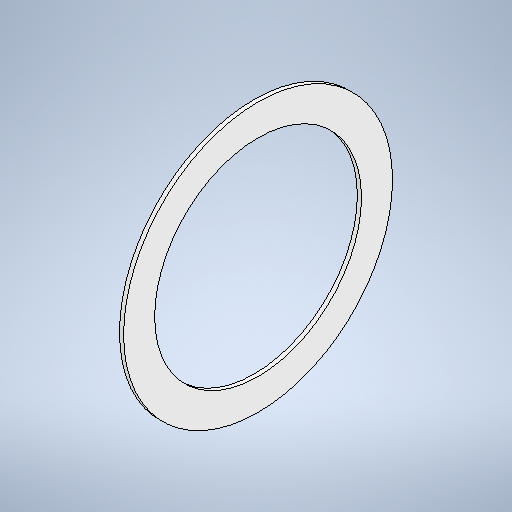
# Autodesk Inventor part: joint4_axis3_washer_2
Saved by Autodesk Inventor 2025.3 (Build 293356030, 356C)
## iProperties
Created: 2025-11-10
Part Number: joint4_axis3_washer_2
Material: PLA filament
Document SubType Name: Modeling
Designer: MSI
Mass: 1.62577 g
Surface Area: 30.7091 cm^2
Volume: 1.35481 cm^3
Density: 1.2 g/cm^3
Appearance: 일반
Author: MSI
Autodesk Inventor part; units mm, degrees
ref_plane "YZ Plane" through (0, 0, 0) normal (1, 0, 0) x (0, 1, 0)
ref_plane "XZ Plane" through (0, 0, 0) normal (0, 1, 0) x (-1, 0, 0)
ref_plane "XY Plane" through (0, 0, 0) normal (0, 0, 1) x (1, 0, 0)
sketch "스케치1" plane through (0, 0, 0) normal (1, 0, 0) x (0, 1, 0)
  circle A0 centre (0, 0) radius 32.5
  circle A1 centre (0, 0) radius 25
  dimension "d0" = 65
  dimension "d1" = 50
  constraints: 2 centre point, 1 coincident
  measures "d0" diameter of A0
  measures "d1" diameter of A1
extrude "돌출1" add sketch "스케치1" along normal mid plane 1
equation "\"d1\" = joint4_axis3_d2"
equation "\"joint4_belt_centor\" = 157.367"
equation "\"joint4_axis2_L\" = 58.803"
equation "\"joint4_axis2_b1\" = 35"
equation "\"joint4_axis2_d\" = 19"
equation "\"joint4_miter_m\" = 2"
equation "\"joint4_miter_a\" = 20deg"
equation "\"joint4_miter_z\" = 79"
equation "\"joint4_miter_b\" = 6.90139"
equation "\"joint4_axis3_L\" = 23.5"
equation "\"joint4_axis3_d2\" = 50"
equation "\"joint3_belt_centor\" = 157.367"
equation "\"joint3_axis2_L\" = 16"
equation "\"joint3_axis2_d\" = 19"
equation "\"joint3_planetary_m\" = 1.5"
equation "\"joint3_planetary_a\" = 20deg"
equation "\"joint3_planetary_np\" = 4"
equation "\"joint3_sun_z\" = 18"
equation "\"joint3_sun_b\" = 17"
equation "\"joint3_planet_z\" = 36"
equation "\"joint3_planet_b\" = 17"
equation "\"joint3_ring_b\" = 9"
equation "\"joint3_axis3_d\" = 29"
equation "\"joint3_miter_m\" = 5.5"
equation "\"joint3_miter_a\" = 20deg"
equation "\"joint3_miter_z\" = 28"
equation "\"joint3_miter_b\" = 13.65957"
equation "\"joint3_axis4_L\" = 23.5"
